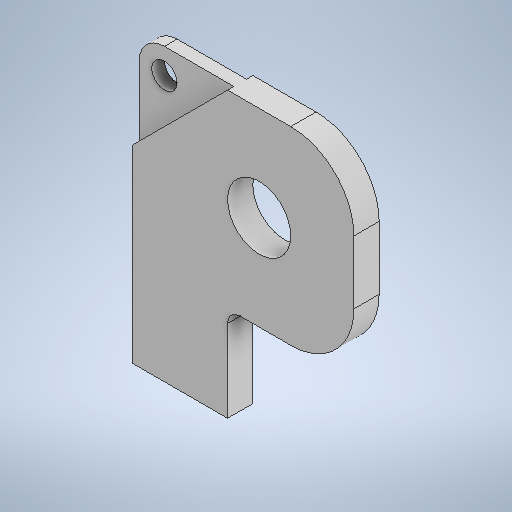
# Autodesk Inventor part: Letra-P-Metalica
Saved by Autodesk Inventor 2025 (Build 290162010, 162A)
## iProperties
Created: 2025-10-14
Part Number: Letra-P-Metalica
Material: Genérico
Document SubType Name: Modeling
Designer: 202321250026
Density: 1 g/cm^3
Appearance: Padrão
Author: 202321250026
Autodesk Inventor part; units mm, degrees
ref_plane "YZ Plane" through (0, 0, 0) normal (1, 0, 0) x (0, 1, 0)
ref_plane "XZ Plane" through (0, 0, 0) normal (0, 1, 0) x (-1, 0, 0)
ref_plane "XY Plane" through (0, 0, 0) normal (0, 0, 1) x (1, 0, 0)
sketch "Esboço7" plane through (0, 0, 0) normal (0, 0, 1) x (1, 0, 0)
  line L0 (-21.4474, -16.1404) -> (-36.4474, -16.1404)
  line L1 (-36.4474, -16.1404) -> (-36.4474, 28.8596)
  line L2 (-36.4474, 28.8596) -> (-1.4474, 28.8596)
  line L3 (-1.4474, 28.8596) -> (-1.4474, -1.1404)
  line L4 (-1.4474, -1.1404) -> (-21.4474, -1.1404)
  line L5 (-21.4474, -1.1404) -> (-21.4474, -16.1404)
  point P0 (0, 0)
  dimension "d28" = 45
  dimension "d29" = 35
  dimension "d30" = 15
  dimension "d31" = 30
  constraints: 12 end point, 5 perpendicular, 1 horizontal
  measures "d28" distance between parallel lines of L0 L2
  measures "d29" distance between parallel lines of L3 L1
  measures "d30" distance between parallel lines of L5 L1
  measures "d31" distance from line of L2 L4.end
extrude "Extrusão2" add sketch "Esboço7" along normal blind 4
fillet "Arredondamento13" radius 4 1 edges at (-36.4474, 28.8596, 2)
fillet "Arredondamento14" radius 10 1 edges at (-1.4474, 28.8596, 2)
fillet "Arredondamento15" radius 10 1 edges at (-1.4474, -1.1404, 2)
fillet "Arredondamento16" radius 2 1 edges at (-21.4474, -1.1404, 2)
sketch "Esboço9" plane through (0, 0, 4) normal (0, 0, 1) x (1, 0, 0)
  arc A0 (-11.4474, -1.1404) -> (-1.4474, 8.8596) centre (-11.4474, 8.8596) ccw projected
  line L0 (-1.4474, 8.8596) -> (-1.4474, 18.8596) projected
  arc A1 (-1.4474, 18.8596) -> (-11.4474, 28.8596) centre (-11.4474, 18.8596) ccw projected
  line L1 (-11.4474, 28.8596) -> (-32.4474, 28.8596) projected
  arc A2 (-32.4474, 28.8596) -> (-36.4474, 24.8596) centre (-32.4474, 24.8596) ccw projected
  line L2 (-36.4474, 24.8596) -> (-36.4474, -16.1404) projected
  line L3 (-36.4474, -16.1404) -> (-21.4474, -16.1404) projected
  line L4 (-21.4474, -16.1404) -> (-21.4474, -3.1404) projected
  arc A3 (-19.4474, -1.1404) -> (-21.4474, -3.1404) centre (-19.4474, -3.1404) ccw projected
  line L5 (-19.4474, -1.1404) -> (-11.4474, -1.1404) projected
  point P0 (0, 0)
  constraints: 1 coincident
hole "Furo3" at (-32.4474, 24.8596, 4) direction (0, 0, -1) diameter 4 end through all
sketch "Esboço10" plane through (0, 0, 4) normal (0, 0, 1) x (1, 0, 0)
  circle A0 centre (-32.4474, 24.8596) radius 2 projected
  arc A1 (-11.4474, -1.1404) -> (-1.4474, 8.8596) centre (-11.4474, 8.8596) ccw projected
  line L0 (-1.4474, 8.8596) -> (-1.4474, 18.8596) projected
  arc A2 (-1.4474, 18.8596) -> (-11.4474, 28.8596) centre (-11.4474, 18.8596) ccw projected
  line L1 (-11.4474, 28.8596) -> (-32.4474, 28.8596) projected
  arc A3 (-32.4474, 28.8596) -> (-36.4474, 24.8596) centre (-32.4474, 24.8596) ccw projected
  line L2 (-36.4474, 24.8596) -> (-36.4474, -16.1404) projected
  line L3 (-36.4474, -16.1404) -> (-21.4474, -16.1404) projected
  line L4 (-21.4474, -16.1404) -> (-21.4474, -3.1404) projected
  arc A4 (-19.4474, -1.1404) -> (-21.4474, -3.1404) centre (-19.4474, -3.1404) ccw projected
  line L5 (-19.4474, -1.1404) -> (-11.4474, -1.1404) projected
  point P0 (0, 0)
  point P1 (-16.4474, 13.8596)
  point P2 (-1.4474, 13.8596)
  point P3 (-16.4474, 13.8596)
  dimension "d52" = 15
  dimension "d53" = 15
  constraints: 1 coincident, 1 midpoint
  measures "d52" distance from line of L5 point (-16.447, 13.86)
  measures "d53" distance of point (-1.447, 13.86) point (-16.447, 13.86)
hole "Furo4" at (-16.4474, 13.8596, 4) direction (0, 0, -1) diameter 10 end through all
sketch "Esboço12" plane through (0, 0, 4) normal (0, 0, 1) x (1, 0, 0)
  circle A0 centre (-16.4474, 13.8596) radius 5 projected
  circle A1 centre (-32.4474, 24.8596) radius 2 projected
  arc A2 (-11.4474, -1.1404) -> (-1.4474, 8.8596) centre (-11.4474, 8.8596) ccw projected
  line L0 (-1.4474, 8.8596) -> (-1.4474, 18.8596) projected
  arc A3 (-1.4474, 18.8596) -> (-11.4474, 28.8596) centre (-11.4474, 18.8596) ccw projected
  line L1 (-11.4474, 28.8596) -> (-32.4474, 28.8596) projected
  arc A4 (-32.4474, 28.8596) -> (-36.4474, 24.8596) centre (-32.4474, 24.8596) ccw projected
  line L2 (-36.4474, 24.8596) -> (-36.4474, -16.1404) projected
  line L3 (-36.4474, -16.1404) -> (-21.4474, -16.1404) projected
  line L4 (-21.4474, -16.1404) -> (-21.4474, -3.1404) projected
  arc A5 (-19.4474, -1.1404) -> (-21.4474, -3.1404) centre (-19.4474, -3.1404) ccw projected
  line L5 (-19.4474, -1.1404) -> (-11.4474, -1.1404) projected
  line L6 (-11.4474, 28.8596) -> (-32.4474, 28.8596) projected
  line L7 (-36.4474, 24.8596) -> (-36.4474, -16.1404) projected
  line L8 (-36.4474, 13.8596) -> (-21.4474, 28.8596)
  point P0 (0, 0)
  constraints: 2 end point, 2 point on line
extrude "Extrusão3" cut sketch "Esboço12" against normal blind 1 contours L8 L2 A4 L1
sketch "Esboço14" plane through (0, 0, 0) normal (0, 0, -1) x (-1, 0, 0)
  circle A0 centre (16.4474, 13.8596) radius 5 projected
  circle A1 centre (32.4474, 24.8596) radius 2 projected
  arc A2 (1.4474, 8.8596) -> (11.4474, -1.1404) centre (11.4474, 8.8596) ccw projected
  line L0 (19.4474, -1.1404) -> (11.4474, -1.1404) projected
  arc A3 (21.4474, -3.1404) -> (19.4474, -1.1404) centre (19.4474, -3.1404) ccw projected
  line L1 (21.4474, -16.1404) -> (21.4474, -3.1404) projected
  line L2 (36.4474, -16.1404) -> (21.4474, -16.1404) projected
  line L3 (36.4474, 24.8596) -> (36.4474, -16.1404) projected
  arc A4 (36.4474, 24.8596) -> (32.4474, 28.8596) centre (32.4474, 24.8596) ccw projected
  line L4 (11.4474, 28.8596) -> (32.4474, 28.8596) projected
  arc A5 (11.4474, 28.8596) -> (1.4474, 18.8596) centre (11.4474, 18.8596) ccw projected
  line L5 (1.4474, 8.8596) -> (1.4474, 18.8596) projected
  line L6 (21.4474, 28.8596) -> (36.4474, 13.8596)
  point P0 (0, 0)
  constraints: 2 end point, 2 point on line
extrude "Extrusão4" cut sketch "Esboço14" against normal blind 1 contours L4 A4 L3 L6
